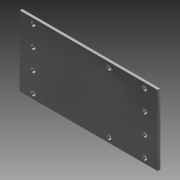
# Autodesk Inventor part: Part77
Saved by Autodesk Inventor 2015 (Build 190159000, 159)
## iProperties
Created: 2015-01-11
Part Number: Part77
Material: Generic
Document SubType Name: Modeling
Designer: mastkee16
Density: 1 g/cm^3
Appearance: Knurled 45
Author: mastkee16
Autodesk Inventor part; units mm, degrees
ref_plane "YZ Plane" through (0, 0, 0) normal (1, 0, 0) x (0, 1, 0)
ref_plane "XZ Plane" through (0, 0, 0) normal (0, 1, 0) x (-1, 0, 0)
ref_plane "XY Plane" through (0, 0, 0) normal (0, 0, 1) x (1, 0, 0)
sketch "Sketch1" plane through (0, 0, 0) normal (0, 0, 1) x (1, 0, 0)
  line L0 (0, 0) -> (174.7774, 0)
  line L1 (174.7774, 0) -> (174.7774, 88.9)
  line L2 (174.7774, 88.9) -> (0, 88.9)
  line L3 (0, 88.9) -> (0, 0)
  dimension "d0" = 174.7774
  dimension "d1" = 88.9
  constraints: 8 end point, 2 parallel, 1 horizontal, 1 perpendicular
  measures "d0" distance of L2.end L1.end
  measures "d1" distance of L1.end L0.end
extrude "Extrusion1" add sketch "Sketch1" along normal blind 3.175
sketch "Sketch2" plane through (0, 0, 3.175) normal (0, 0, 1) x (1, 0, 0)
  line L0 (174.7774, 88.9) -> (0, 88.9) projected
  line L1 (0, 0) -> (174.7774, 0) projected
  line L2 (174.7774, 0) -> (174.7774, 88.9) projected
  line L3 (0, 88.9) -> (0, 0) projected
  point P0 (16.8148, 82.55)
  point P1 (16.8148, 57.15)
  point P2 (157.9626, 57.15)
  point P3 (157.9626, 82.55)
  point P4 (16.8148, 31.75)
  point P5 (157.9626, 31.75)
  point P6 (157.9626, 6.35)
  point P7 (16.8148, 6.35)
  dimension "d4" = 6.35
  dimension "d5" = 25.4
  dimension "d6" = 88.9
  dimension "d7" = 6.35
  dimension "d8" = 25.4
  dimension "d9" = 16.8148
  dimension "d10" = 16.8148
  dimension "d11" = 16.8148
  dimension "d12" = 16.8148
  dimension "d31" = 25.4
  dimension "d32" = 25.4
  dimension "d33" = 25.4
  dimension "d34" = 25.4
  measures "d4" distance from line of L0 point (16.815, 82.55)
  measures "d5" distance of point (16.815, 82.55) point (16.815, 57.15)
  measures "d6" distance between parallel lines of L1 L0
  measures "d7" distance from line of L0 point (157.963, 82.55)
  measures "d8" distance of point (157.963, 57.15) point (157.963, 82.55)
  measures "d9" distance from line of L2 point (157.963, 57.15)
  measures "d10" distance from line of L2 point (157.963, 82.55)
  measures "d11" distance from line of L3 point (16.815, 82.55)
  measures "d12" distance from line of L3 point (16.815, 57.15)
  measures "d31" distance of point (16.815, 31.75) point (16.815, 57.15)
  measures "d32" distance of point (157.963, 31.75) point (157.963, 57.15)
  measures "d33" distance of point (157.963, 6.35) point (157.963, 31.75)
  measures "d34" distance of point (16.815, 6.35) point (16.815, 31.75)
hole "Hole1" at (16.8148, 82.55, 3.175) at (16.8148, 57.15, 3.175) at (157.9626, 57.15, 3.175) at (157.9626, 82.55, 3.175) at (16.8148, 31.75, 3.175) at (16.8148, 6.35, 3.175) at (157.9626, 6.35, 3.175) at (157.9626, 31.75, 3.175) direction (0, 0, -1) diameter 6.35 end through all
sketch "Sketch3" plane through (0, 0, 3.175) normal (0, 0, 1) x (1, 0, 0)
  line L0 (0, 88.9) -> (0, 0) projected
  line L1 (174.7774, 88.9) -> (0, 88.9) projected
  line L2 (0, 0) -> (174.7774, 0) projected
  point P0 (112.7887, 82.55)
  point P1 (112.7887, 6.35)
  dimension "d20" = 112.7887
  dimension "d21" = 112.7887
  dimension "d22" = 6.35
  dimension "d23" = 6.35
  measures "d20" distance from line of point (112.789, 82.55) L0
  measures "d21" distance from line of point (112.789, 6.35) L0
  measures "d22" distance from line of L1 point (112.789, 82.55)
  measures "d23" distance from line of L2 point (112.789, 6.35)
hole "Hole2" at (112.7887, 82.55, 3.175) at (112.7887, 6.35, 3.175) direction (0, 0, -1) diameter 6.35 end through all
body "Solid1"
